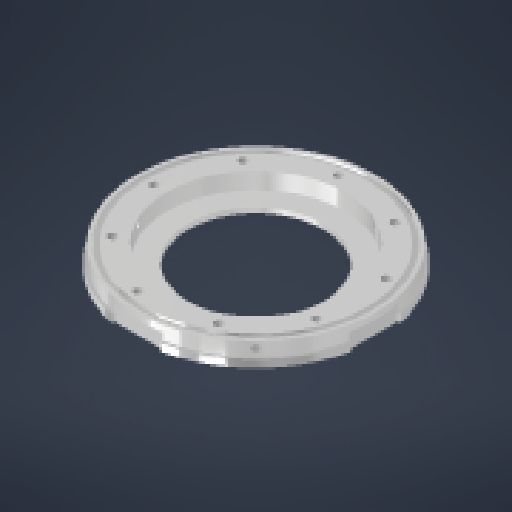
# Autodesk Inventor part: Ring_unten
Saved by Autodesk Inventor 2027 (Build 310192060, 192F)
## iProperties
Created: 2026-08-01
Part Number: Ring_unten
Material: Aluminum 6061
Document SubType Name: Modeling
Designer: kw
Density: 2.7 g/cm^3
Appearance: Aluminum - Flat
Author: kw
Autodesk Inventor part; units mm, degrees
note: some values were not read from the file. Chosen so that the rebuilt part matches the saved one: direction of "Hole2"; pattern direction of "Circular Pattern2".
ref_plane "XZ Plane" through (0, 0, 0) normal (0, 1, 0) x (-1, 0, 0)
sketch "Sketch1" plane through (0, 0, 0) normal (0, 1, 0) x (-1, 0, 0)
  circle A0 centre (0, 0) radius 47
  circle A1 centre (0, 0) radius 26.5
  circle A2 centre (0, 0) radius 35
  dimension "d0" = 94
  dimension "d1" = 53
  dimension "d2" = 70
  constraints: 3 centre point, 3 coincident
  measures "d0" diameter of A0
  measures "d1" diameter of A1
  measures "d2" diameter of A2
extrude "Extrusion1" add sketch "Sketch1" along normal blind 2 contours A2
extrude "Extrusion2" add sketch "Sketch1" along normal blind 8.5 contours A0
sketch "Sketch2" plane through (0, 8.5, 0) normal (0, 1, 0) x (1, 0, 0)
  circle A0 centre (0, 0) radius 40
  point P0 (-40, 0)
  point P1 (-30.6418, -25.7115)
  point P2 (-6.9459, -39.3923)
  point P3 (20, -34.641)
  point P4 (37.5877, -13.6808)
  point P5 (37.5877, 13.6808)
  point P6 (20, 34.641)
  point P7 (-6.9459, 39.3923)
  point P8 (-30.6418, 25.7115)
  dimension "d10" = 80
  dimension "d13" = 360
  constraints: 1 coincident, 1 horizontal alignment, 12 other
hole "Hole1" at (-40, 8.5, 0) at (-30.6418, 8.5, 25.7115) at (-6.9459, 8.5, 39.3923) at (20, 8.5, 34.641) at (37.5877, 8.5, 13.6808) at (37.5877, 8.5, -13.6808) at (20, 8.5, -34.641) at (-6.9459, 8.5, -39.3923) at (-30.6418, 8.5, -25.7115) direction (0, -1, 0) diameter 3.242 end through all thread size "M4x0.7" class "6H" standard "ISO Metric profile"
ref_plane "Work Plane1" through (47, 0, 0) normal (1, 0, 0) x (0, 1, 0)
sketch "Sketch3" plane through (47, 0, 0) normal (1, 0, 0) x (0, 1, 0)
  line L0 (0, 26.5) -> (0, -26.5) projected
  line L1 (8.5, -47) -> (8.5, 47) projected
  line L2 (0, 2.5) -> (8.5, 2.5)
  line L3 (8.5, 2.5) -> (8.5, -2.5)
  line L4 (8.5, -2.5) -> (0, -2.5)
  line L5 (0, -2.5) -> (0, 2.5)
  line L6 (0, 10) -> (8.5, 10)
  line L7 (8.5, 10) -> (8.5, -10)
  line L8 (8.5, -10) -> (0, -10)
  line L9 (0, -10) -> (0, 10)
  line L10 (6, 10) -> (6, -10)
  point P0 (0, 0)
  dimension "d23" = 5
  dimension "d26" = 20
  constraints: 18 end point, 6 point on line, 4 parallel, 3 perpendicular, 2 horizontal
  measures "d23" distance of L2.end L3.end
  measures "d26" distance of L6.end L7.end
extrude "Extrusion4" cut sketch "Sketch3" against normal blind 1 contours L6 L10 L2 L0 | L2 L10 L4 L0 | L4 L10 L8 L0
pattern_circular "Circular Pattern1" count 4 over 360 about axis through (0, 0, 0) along (0, 1, 0) of "Extrusion4"
sketch "Sketch4" plane through (0, 8.5, 0) normal (0, 1, 0) x (1, 0, 0)
  circle A0 centre (20, 34.641) radius 1.621 projected
  circle A1 centre (0, 0) radius 42
  circle A2 centre (0, 0) radius 47
  circle A3 centre (0, 0) radius 43.5
  circle A4 centre (0, 0) radius 45.5
  dimension "d31" = 84
  dimension "d33" = 94
  dimension "d34" = 87
  dimension "d35" = 91
  constraints: 4 centre point, 3 coincident
  measures "d31" diameter of A1
  measures "d33" diameter of A2
  measures "d34" diameter of A3
  measures "d35" diameter of A4
extrude "Extrusion5" cut sketch "Sketch4" against normal blind 1 contours A4
sketch "Sketch5" plane through (0, 0, 0) normal (0, 1, 0) x (-1, 0, 0)
  line L0 (0, 0) -> (-35.3553, 35.3553)
  line L1 (0, 0) -> (50, 0) construction
  dimension "d38" = 50
  dimension "d39" = 135
  constraints: 4 end point, 1 equal length, 1 horizontal
  measures "d38" distance of L0.start L0.end
  measures "d39" angle of L1 L0
ref_plane "Work Plane2" through (33.234, 0, 33.234) normal (0.7071068, 0, 0.7071068) x (0, 1, 0)
sketch "Sketch6" plane through (33.234, 0, 33.234) normal (0.7071068, 0, 0.7071068) x (0, 1, 0)
  point P0 (0, 0)
  point P1 (6, 0)
hole "Hole2" at (33.234, 6, 33.234) direction (-0.7071068, 0, -0.7071068) diameter 2.459 end up to surface thread size "M3x0.5" class "6H" standard "ISO Metric profile"
pattern_circular "Circular Pattern2" count 3 over 220 about axis through (0, 0, 0) along (0, 1, 0) of "Hole2" both ways yes
sketch "Sketch7" plane through (0, 0, 0) normal (0, -1, 0) x (1, 0, 0)
  circle A0 centre (0, 0) radius 47
  circle A1 centre (0, 0) radius 48
  line L0 (0, 0) -> (9.8488, 46.9787)
  line L1 (0, 0) -> (-9.8488, 46.9787)
  line L2 (0, 0) -> (-46.9787, -9.8488)
  line L3 (0, 0) -> (-46.9787, 9.8488)
  line L4 (0, 0) -> (9.8488, -46.9787)
  line L5 (0, 0) -> (-9.8488, -46.9787)
  line L6 (0, 0) -> (46.9787, 9.8488)
  line L7 (0, 0) -> (46.9787, -9.8488)
  point P0 (-46, 9.6437)
  point P1 (-9.6437, 46)
  point P2 (46, 9.6437)
  point P3 (9.6437, 46)
  point P4 (46, -9.6437)
  point P5 (9.6437, -46)
  point P6 (-9.6437, -46)
  point P7 (-46, -9.6437)
  dimension "d53" = 1
  dimension "d54" = 48
  dimension "d55" = 48
  dimension "d58" = 360
  constraints: 16 end point, 3 coincident, 2 centre point, 19 other
  measures "d53" radial gap between concentric circles of A0 A1
  measures "d54" distance of L0.start L0.end
  measures "d55" distance of L0.start L1.end
extrude "Extrusion6" add sketch "Sketch7" against normal blind 3 contours A0 L0 A1 L6 | L7 A1 L4 A0 | A0 L3 A1 L1 | A0 L5 A1 L2
body "Solid1"
